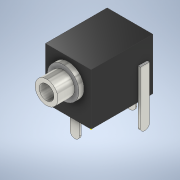
# Autodesk Inventor part: PY-401N
Saved by Autodesk Inventor 2020 (Build 240168000, 168)
## iProperties
Created: 2021-05-20
Part Number: PY-401N
Material: Типовые
Document SubType Name: Modeling
Designer: Михаил
Density: 1 g/cm^3
Appearance: По умолчанию
Author: Михаил
Autodesk Inventor part; units mm, degrees
ref_plane "YZ Plane" through (0, 0, 0) normal (1, 0, 0) x (0, 1, 0)
ref_plane "XZ Plane" through (0, 0, 0) normal (0, 1, 0) x (-1, 0, 0)
ref_plane "XY Plane" through (0, 0, 0) normal (0, 0, 1) x (1, 0, 0)
sketch "Эскиз1" plane through (0, 0, 0) normal (0, 1, 0) x (-1, 0, 0)
  line L0 (0, 0) -> (8, 0)
  line L1 (8, 0) -> (8, -10.8)
  line L2 (8, -10.8) -> (0, -10.8)
  line L3 (0, -10.8) -> (0, 0)
  dimension "d0" = 10.8
  dimension "d1" = 8
  constraints: 8 end point, 2 parallel, 1 horizontal, 1 perpendicular
  measures "d0" distance of L0.end L1.end
  measures "d1" distance of L1.end L2.end
extrude "Выдавливание1" add sketch "Эскиз1" along normal blind 9
sketch "Эскиз2" plane through (-8, 0, 0) normal (0, 0, 1) x (1, 0, 0)
  circle A0 centre (4, 5.5) radius 2.75
  line L0 (8, 0) -> (8, 9) projected
  line L1 (0, 0) -> (8, 0) projected
  dimension "d4" = 5.5
  dimension "d5" = 4
  dimension "d6" = 5.5
  constraints: 1 centre point
  measures "d4" diameter of A0
  measures "d5" distance from line of L0 A0.centre
  measures "d6" distance from line of L1 A0.centre
extrude "Выдавливание2" add sketch "Эскиз2" along normal blind 0.9
sketch "Эскиз3" plane through (-4, 5.5, 0.9) normal (0, 0, 1) x (1, 0, 0)
  circle A0 centre (0, 0) radius 2
  point P0 (4, -5.5)
  dimension "d9" = 4
  constraints: 1 centre point
  measures "d9" diameter of A0
extrude "Выдавливание3" add sketch "Эскиз3" along normal blind 2.9
sketch "Эскиз4" plane through (-4, 5.5, 3.8) normal (0, 0, 1) x (1, 0, 0)
  circle A0 centre (0, 0) radius 2.75 projected
  circle A1 centre (0, 0) radius 1.275
  point P0 (4, -5.5)
  dimension "d12" = 2.55
  constraints: 1 centre point, 1 coincident
  measures "d12" diameter of A1
extrude "Выдавливание4" cut sketch "Эскиз4" against normal blind 7.9 contours A1
sketch "Эскиз5" plane through (-8, 0, 0) normal (0, 0, 1) x (1, 0, 0)
  point P0 (8, 0)
sketch "Эскиз6" plane through (0, 0, 0) normal (0, -1, 0) x (1, 0, 0)
  line L0 (-4.8, -1.15) -> (-3.2, -1.15)
  line L1 (-3.2, -1.15) -> (-3.2, -1.45)
  line L2 (-3.2, -1.45) -> (-4.8, -1.45)
  line L3 (-4.8, -1.45) -> (-4.8, -1.15)
  line L4 (0, 0) -> (0, -10.8) projected
  line L5 (-8, 0) -> (0, 0) projected
  dimension "d15" = 1.6
  dimension "d16" = 0.3
  dimension "d17" = 3.2
  dimension "d18" = 1.15
  constraints: 8 end point, 2 parallel, 1 horizontal, 1 perpendicular
  measures "d15" distance of L1.end L2.end
  measures "d16" distance of L0.end L1.end
  measures "d17" distance between parallel lines of L4 L1
  measures "d18" distance between parallel lines of L0 L5
extrude "Выдавливание5" add sketch "Эскиз6" along normal blind 4
sketch "Эскиз7" plane through (-4.8, 0, -1.15) normal (0, 0, 1) x (1, 0, 0)
  line L0 (0, 0) -> (0, -4) projected
  line L1 (1.6, 0) -> (1.6, -4) projected
  arc A0 (0, -3.2011) -> (1.6, -3.2011) centre (0.8, -3.2011) ccw
  line L2 (0, -3.2011) -> (0, -4)
  line L3 (1.6, -4) -> (0, -4) projected
  line L4 (1.6, -4) -> (1.6, -3.2011)
  point P0 (4.8, 0)
  point P1 (0.7588, -4)
  point P2 (0.8412, -4)
  constraints: 4 end point, 2 point on circle, 2 point on line, 2 tangent, 1 centre point, 1 collinear, 1 parallel
extrude "Выдавливание6" cut sketch "Эскиз7" against normal blind 4
sketch "Эскиз8" plane through (0, 0, 0) normal (1, 0, 0) x (0, 0, -1)
  line L0 (8.2, 5.5) -> (9.8, 5.5)
  line L1 (9.8, 5.5) -> (9.8, -4.5)
  line L2 (9.8, -4.5) -> (8.2, -4.5)
  line L3 (8.2, -4.5) -> (8.2, 5.5)
  line L4 (0, 9) -> (10.8, 9) projected
  line L5 (0, 0) -> (0, 9) projected
  dimension "d23" = 1.6
  dimension "d24" = 3.5
  dimension "d25" = 8.2
  dimension "d26" = 10
  constraints: 8 end point, 2 parallel, 1 horizontal, 1 perpendicular
  measures "d23" distance of L1.end L2.end
  measures "d24" distance between parallel lines of L4 L0
  measures "d25" distance between parallel lines of L5 L3
  measures "d26" distance of L0.end L1.end
extrude "Выдавливание7" add sketch "Эскиз8" along normal blind 0.4
sketch "Эскиз9" plane through (0.4, 0, 0) normal (1, 0, 0) x (0, 0, -1)
  line L0 (8.2, 0) -> (8.2, -4.5) projected
  line L1 (9.8, -4.5) -> (9.8, 0) projected
  arc A0 (8.2, -3.8439) -> (9.8, -3.8337) centre (8.999, -3.6854) ccw
  line L2 (8.2, -3.8439) -> (8.2, -4.5)
  line L3 (8.2, -4.5) -> (9.8, -4.5) projected
  line L4 (9.8, -4.5) -> (9.8, -3.8337)
  point P0 (0, 0)
  point P1 (8.9981, -4.5)
  constraints: 4 end point, 2 point on circle, 2 point on line, 1 centre point, 1 collinear, 1 parallel
extrude "Выдавливание8" cut sketch "Эскиз9" against normal blind 0.4
sketch "Эскиз10" plane through (0, 0, -10.8) normal (0, 0, -1) x (-1, 0, 0)
  line L0 (3, 0.35) -> (5, 0.35)
  line L1 (5, 0.35) -> (5, -4.4)
  line L2 (5, -4.4) -> (3, -4.4)
  line L3 (3, -4.4) -> (3, 0.35)
  line L4 (8, 0) -> (8, 9) projected
  line L5 (0, 0) -> (8, 0) projected
  dimension "d31" = 2
  dimension "d32" = 3
  dimension "d33" = 4.75
  dimension "d34" = 0.35
  constraints: 8 end point, 2 parallel, 1 horizontal, 1 perpendicular
  measures "d31" distance of L1.end L2.end
  measures "d32" distance between parallel lines of L4 L1
  measures "d33" distance of L2.end L0.start
  measures "d34" distance between parallel lines of L5 L0
extrude "Выдавливание9" add sketch "Эскиз10" along normal blind 0.2
sketch "Эскиз11" plane through (0, 0, -11) normal (0, 0, -1) x (-1, 0, 0)
  line L0 (3, 0.35) -> (3, -4.4) projected
  line L1 (5, -4.4) -> (5, 0.35) projected
  arc A0 (3, -3.4779) -> (5, -3.4779) centre (4, -3.3967) ccw
  line L2 (3, -4.4) -> (5, -4.4) projected
  line L3 (3, -3.4779) -> (3, -4.4)
  line L4 (3, -4.4) -> (5, -4.4)
  line L5 (5, -4.4) -> (5, -3.4779)
  point P0 (0, 0)
  point P1 (4, -4.4)
  constraints: 6 end point, 2 collinear, 2 point on circle, 2 point on line, 1 centre point, 1 perpendicular
extrude "Выдавливание10" cut sketch "Эскиз11" against normal blind 0.2
